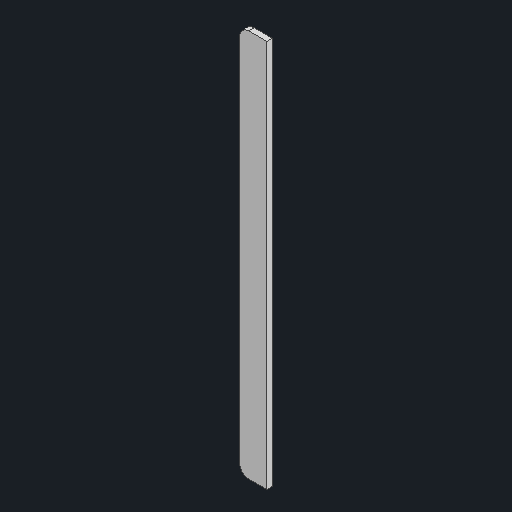
# Autodesk Inventor part: DMF 2.1 Пластина паза маленькая
Saved by Autodesk Inventor 2026.2 (Build 302298010, 298A)
## iProperties
Created: 2024-04-30
Part Number: DMF 2.1 Пластина паза маленькая
Material: Generic
Document SubType Name: Sheet Metal
Designer: pokla
Stock Number: DMF 2.1 Пластина паза маленькая
Density: 1 g/cm^3
Sheet Metal Rule: Default
Sheet Metal Width: 212,492 mm
Sheet Metal Length: 15,000 mm
Sheet Metal Area: 3187,380 mm^2
Appearance: Default
Flat Pattern Width: 21.2492 cm
Flat Pattern Length: 1.5 cm
Flat Pattern Area: 31.8738 cm^2
Author: pokla
Autodesk Inventor part; units mm, degrees
ref_plane "YZ Plane" through (0, 0, 0) normal (1, 0, 0) x (0, 1, 0)
ref_plane "XZ Plane" through (0, 0, 0) normal (0, 1, 0) x (-1, 0, 0)
ref_plane "XY Plane" through (0, 0, 0) normal (0, 0, 1) x (1, 0, 0)
sketch "Sketch1" plane through (0, 0, 0) normal (0, 0, 1) x (1, 0, 0)
  line L0 (-7.5, 212.492) -> (7.5, 212.492)
  line L1 (7.5, 212.492) -> (7.5, 0)
  line L2 (7.5, 0) -> (-7.5, 0)
  line L3 (-7.5, 0) -> (-7.5, 212.492)
  point P0 (0, 0)
  point P1 (0, 0)
  point P2 (0, 0)
  point P3 (0, 0)
  point P4 (0, 0)
  dimension "d27" = 15
  dimension "d29" = 212.492
  measures "d27" distance of L1.end L2.end
  measures "d29" distance between parallel lines of L2 L0
extrude "Plate1" add sketch "Sketch1" along normal mid plane 3
fillet "Fillet2" radius 5 2 edges at (-7.5, 212.492, 0) (-7.5, 0, 0)
equation "\"d15\" = Thickness"
equation "\"BendRadius\" = Thickness"
equation "\"BendReliefWidth\" = Thickness"
equation "\"BendReliefDepth\" = 0.5 * Thickness"
equation "\"CornerReliefSize\" = 4 * Thickness"
equation "\"MinimumRemnant\" = 2 * Thickness"
equation "\"TransitionRadius\" = BendRadius"
equation "\"JacobiRadiusSize\" = BendRadius"
equation "\"GapSize\" = Thickness"
equation "\"Thickness\" = 3"
body "Solid1"
